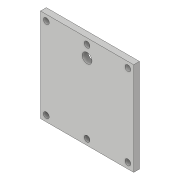
# Autodesk Inventor part: 2 nd part of capping syatem
Saved by Autodesk Inventor 2019 (Build 230136000, 136)
## iProperties
Created: 2019-10-12
Part Number: 2 nd part of capping syatem
Material: Generic
Document SubType Name: Modeling
Designer: Admin
Density: 1 g/cm^3
Appearance: Default
Author: Admin
Autodesk Inventor part; units mm, degrees
ref_plane "YZ Plane" through (0, 0, 0) normal (1, 0, 0) x (0, 1, 0)
ref_plane "XZ Plane" through (0, 0, 0) normal (0, 1, 0) x (-1, 0, 0)
ref_plane "XY Plane" through (0, 0, 0) normal (0, 0, 1) x (1, 0, 0)
sketch "Sketch1" plane through (0, 0, 0) normal (0, 0, 1) x (1, 0, 0)
  line L0 (0, 0) -> (160, 0)
  line L1 (160, 0) -> (160, 160)
  line L2 (160, 160) -> (0, 160)
  line L3 (0, 160) -> (0, 0)
  line L4 (0, 160) -> (10, 160)
  dimension "d0" = 160
  dimension "d1" = 160
  constraints: 10 end point, 2 parallel, 1 horizontal, 1 perpendicular, 1 point on line
  measures "d0" distance of L2.end L1.end
  measures "d1" distance of L1.end L0.end
extrude "Extrusion1" add sketch "Sketch1" along normal blind 10
sketch "Sketch2" plane through (0, 0, 10) normal (0, 0, 1) x (1, 0, 0)
  line L0 (0, 0) -> (0, 10)
  line L1 (0, 160) -> (0, 0) projected
  line L2 (0, 10) -> (0, 160)
  line L3 (0, 160) -> (150, 160)
  line L4 (160, 160) -> (0, 160) projected
  line L5 (150, 160) -> (150, 10)
  line L6 (150, 10) -> (0, 10)
  line L7 (0, 10) -> (0, 160)
  line L8 (0, 160) -> (10, 160)
  line L9 (10, 160) -> (10, 10)
  line L10 (10, 10) -> (150, 10)
  line L11 (150, 160) -> (150, 150)
  line L12 (10, 160) -> (10, 150)
  line L13 (10, 150) -> (150, 150)
  circle A0 centre (10, 150) radius 5
  circle A1 centre (150, 150) radius 5
  circle A2 centre (10, 10) radius 5
  circle A3 centre (150, 10) radius 5
  dimension "d4" = 10
  dimension "d5" = 150
  dimension "d6" = 150
  dimension "d7" = 150
  dimension "d8" = 150
  dimension "d9" = 150
  dimension "d10" = 10
  dimension "d11" = 150
  dimension "d12" = 10
  dimension "d13" = 10
  dimension "d14" = 10
  dimension "d15" = 10
  dimension "d16" = 10
  constraints: 24 end point, 6 point on line, 4 centre point, 4 coincident, 2 collinear, 2 perpendicular
  measures "d4" distance of L0.start L0.end
  measures "d5" distance of L0.end L1.start
  measures "d6" distance of L1.start L3.end
  measures "d7" distance of L3.end L5.end
  measures "d8" distance of L5.end L0.end
  measures "d9" distance of L0.end L1.start
  measures "d10" distance of L1.start L8.end
  measures "d11" distance of L8.end L9.end
  measures "d12" distance of L8.end L12.end
  measures "d13" diameter of A0
  measures "d14" diameter of A1
  measures "d15" diameter of A2
  measures "d16" diameter of A3
extrude "Extrusion2" cut sketch "Sketch2" against normal through all contours A2 L9 L6 | L6 A2 | A0 L13 L9 | L9 A0 | L9 A2 L6 | A1 L5 | L5 L13 A1 | L13 A0 L9 | A3 L5 L6 | L6 L5 A3 | L5 A1 L13
sketch "Sketch3" plane through (0, 0, 10) normal (0, 0, 1) x (1, 0, 0)
  line L0 (0, 160) -> (0, 0) projected
  line L1 (0, 0) -> (80, 0)
  line L2 (0, 0) -> (160, 0) projected
  line L3 (80, 0) -> (80, 10)
  line L4 (80, 10) -> (80, 150)
  circle A0 centre (80, 10) radius 5
  circle A1 centre (80, 150) radius 5
  dimension "d19" = 80
  dimension "d20" = 10
  dimension "d21" = 140
  dimension "d22" = 10
  dimension "d23" = 10
  constraints: 6 end point, 2 centre point, 2 coincident, 1 midpoint, 1 perpendicular, 1 point on line
  measures "d19" distance of L0.end L1.end
  measures "d20" distance of L1.end L3.end
  measures "d21" distance of L3.end L4.end
  measures "d22" diameter of A0
  measures "d23" diameter of A1
extrude "Extrusion3" cut sketch "Sketch3" against normal through all
sketch "Sketch4" plane through (0, 0, 10) normal (0, 0, 1) x (1, 0, 0)
  line L0 (160, 160) -> (0, 160) projected
  line L1 (0, 160) -> (80, 160)
  line L2 (80, 160) -> (80, 130)
  circle A0 centre (80, 130) radius 8.5
  point P0 (0, 0)
  dimension "d26" = 80
  dimension "d27" = 30
  dimension "d28" = 17
  constraints: 4 end point, 1 centre point, 1 coincident, 1 midpoint, 1 perpendicular
  measures "d26" distance of L0.end L1.end
  measures "d27" distance of L1.end L2.end
  measures "d28" diameter of A0
extrude "Extrusion4" cut sketch "Sketch4" against normal through all
body "Solid1"
